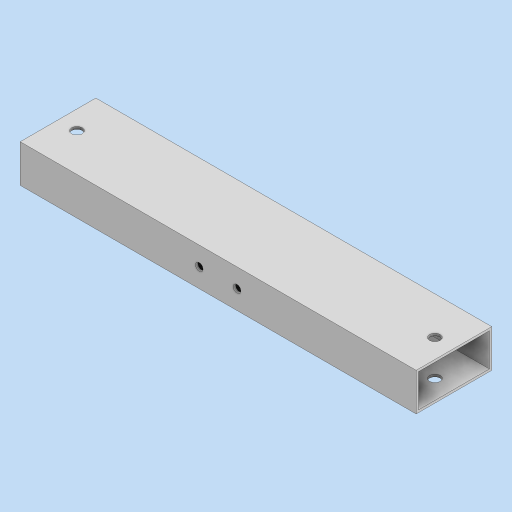
# Autodesk Inventor part: 2inTubeBase
Saved by Autodesk Inventor 2024 (Build 280153000, 153)
## iProperties
Created: 2024-01-10
Part Number: 2inTubeBase
Material: Generic
Document SubType Name: Modeling
Designer: megan
Density: 1 g/cm^3
Appearance: Default
Author: megan
Autodesk Inventor part; units mm, degrees
ref_plane "YZ Plane" through (0, 0, 0) normal (1, 0, 0) x (0, 1, 0)
ref_plane "XZ Plane" through (0, 0, 0) normal (0, 1, 0) x (-1, 0, 0)
ref_plane "XY Plane" through (0, 0, 0) normal (0, 0, 1) x (1, 0, 0)
sketch "Sketch1" plane through (0, 0, 0) normal (1, 0, 0) x (0, 1, 0)
  line L0 (0, 0) -> (25.4, 0)
  line L1 (25.4, 0) -> (25.4, -50.8)
  line L2 (25.4, -50.8) -> (0, -50.8)
  line L3 (0, -50.8) -> (0, 0)
  line L4 (23.8125, -1.5875) -> (1.5875, -1.5875)
  line L5 (1.5875, -1.5875) -> (1.5875, -49.2125)
  line L6 (1.5875, -49.2125) -> (23.8125, -49.2125)
  line L7 (23.8125, -49.2125) -> (23.8125, -1.5875)
  dimension "d0" = 25.4
  dimension "d1" = 50.8
  dimension "d2" = 1.5875
  constraints: 16 end point, 4 parallel, 2 perpendicular, 1 horizontal, 3 other
  measures "d0" distance of L1.end L2.end
  measures "d1" distance of L0.end L1.end
  measures "d2" distance between parallel lines of L0 L4
extrude "Extrusion1" add sketch "Sketch1" along normal blind 266.0208
sketch "Sketch2" plane through (0, 25.4, 0) normal (0, 1, 0) x (1, 0, 0)
  line L0 (0, 50.8) -> (0, 0) projected
  line L1 (0, 0) -> (266.0208, 0) projected
  line L2 (266.0208, 50.8) -> (266.0208, 0) projected
  line L3 (0, 50.8) -> (266.0208, 50.8) projected
  circle A0 centre (12.7, 25.4) radius 3.5687
  circle A1 centre (253.2126, 25.4) radius 3.5687
  point P0 (0, 0)
  dimension "d5" = 7.1374
  dimension "d6" = 12.7
  dimension "d7" = 7.1374
  dimension "d9" = 25.4
  dimension "d10" = 25.4
  dimension "d29" = 240.5126
  constraints: 2 centre point
  measures "d5" diameter of A0
  measures "d6" distance from line of L0 A0.centre
  measures "d7" diameter of A1
  measures "d9" distance from line of A0.centre L3
  measures "d10" distance from line of L1 A1.centre
  measures "d29" distance of A1.centre A0.centre
extrude "Extrusion2" cut sketch "Sketch2" against normal blind 25.4 contours A0 | A1
sketch "Sketch4" plane through (0, 0, 0) normal (0, 0, 1) x (1, 0, 0)
  line L0 (0, 25.4) -> (0, 0) projected
  line L1 (0, 0) -> (266.0208, 0) projected
  line L2 (266.0208, 25.4) -> (266.0208, 0) projected
  line L3 (0, 25.4) -> (266.0208, 25.4) projected
  line L4 (133.0104, 25.4) -> (133.0104, 0) construction
  circle A0 centre (120.3104, 12.7) radius 2.5781
  circle A1 centre (145.7104, 12.7) radius 2.5781
  dimension "d21" = 5.1562
  dimension "d22" = 5.1562
  dimension "d23" = 12.7
  dimension "d24" = 25.4
  dimension "d27" = 12.7
  dimension "d28" = 12.7
  constraints: 2 centre point, 2 end point, 2 midpoint
  measures "d21" diameter of A0
  measures "d22" diameter of A1
  measures "d23" distance from line of L4 A0.centre
  measures "d24" distance of A1.centre A0.centre
  measures "d27" distance from line of L3 A0.centre
  measures "d28" distance from line of L3 A1.centre
extrude "Extrusion4" cut sketch "Sketch4" against normal through all contours A0 | A1
body "Solid1"
